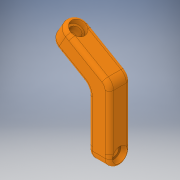
# Autodesk Inventor part: Link2
Saved by Autodesk Inventor 2019 (Build 230136000, 136)
## iProperties
Created: 2022-07-14
Part Number: Link2
Material: Generic
Document SubType Name: Modeling
Designer: zreik
Density: 1 g/cm^3
Appearance: Orange
d46: 10.000 mm
Author: zreik
Autodesk Inventor part; units mm, degrees
ref_plane "YZ Plane" through (0, 0, 0) normal (1, 0, 0) x (0, 1, 0)
ref_plane "XZ Plane" through (0, 0, 0) normal (0, 1, 0) x (-1, 0, 0)
ref_plane "XY Plane" through (0, 0, 0) normal (0, 0, 1) x (1, 0, 0)
sketch "Sketch1" plane through (0, 0, 0) normal (0, 0, 1) x (1, 0, 0)
  line L0 (44.0637, 0) -> (0, 0)
  line L1 (0, 0) -> (34.8308, 60.3287)
  line L2 (34.0637, 0) -> (34.0637, 22.1132)
  line L3 (31.5637, 26.4434) -> (19.3412, 33.5)
  line L4 (44.0637, 0) -> (44.0637, 27.8868)
  line L5 (41.5637, 32.2169) -> (24.3412, 42.1603)
  arc A0 (34.0637, 22.1132) -> (31.5637, 26.4434) centre (29.0637, 22.1132) ccw
  arc A1 (44.0637, 27.8868) -> (41.5637, 32.2169) centre (39.0637, 27.8868) ccw
  line L6 (24.3412, 42.1603) -> (19.3412, 33.5)
  line L7 (24.3412, 42.1603) -> (41.5637, 32.2169)
  line L8 (19.3412, 33.5) -> (31.5637, 26.4434)
  line L9 (34.0637, 0) -> (44.0637, 0)
  line L10 (44.0637, 0) -> (44.0637, 27.8868)
  line L11 (34.0637, 0) -> (44.0637, 0)
  line L12 (44.0637, 0) -> (44.0637, 27.8868)
  line L13 (41.5637, 32.2169) -> (24.3412, 42.1603)
  line L14 (24.3412, 42.1603) -> (19.3412, 33.5)
  line L15 (19.3412, 33.5) -> (31.5637, 26.4434)
  line L16 (34.0637, 22.1132) -> (34.0637, 0)
  point P0 (25, 43.3013)
  point P1 (34.0637, 25)
  dimension "d37" = 60
  dimension "d38" = 10
  dimension "d39" = 10
  dimension "d40" = 0
  dimension "d41" = 0
  dimension "d42" = 25
  dimension "d43" = 17
  dimension "d44" = 120
  dimension "d45" = 5
  constraints: 34 end point, 9 collinear, 6 point on line, 4 point on circle, 4 tangent, 2 centre point, 2 parallel, 1 coincident, 1 equal radius, 1 horizontal, 1 vertical
  measures "d37" angle of L1 L0
  measures "d38" distance between parallel lines of L3 L5
  measures "d39" distance between parallel lines of L4 L2
  measures "d40" distance from line of L1 L3.end
  measures "d41" distance from line of L1 L5.end
  measures "d42" distance of L2.start point (34.064, 25)
  measures "d43" distance of point (34.064, 25) L3.end
  measures "d44" angle of L2 L3
  measures "d45" radius of A0
extrude "Extrusion1" add sketch "Sketch1" along normal blind 10 contours L0 L2 A0 L3 L1 L5 A1 L4
ref_plane "Work Plane1" through (41.5637, 32.2169, 0) normal (0.5, 0.8660254, 0) x (-0.8660254, 0.5, 0)
sketch "Sketch2" plane through (41.5637, 32.2169, 0) normal (0.5, 0.8660254, 0) x (-0.8660254, 0.5, 0)
  circle A0 centre (19.8868, 5) radius 5
  line L0 (19.8868, 0) -> (19.8868, 10) projected
  line L1 (0, 10) -> (19.8868, 10) projected
  dimension "d5" = 10
  dimension "d47" = 0
  dimension "d48" = 5
  constraints: 1 centre point
  measures "d5" diameter of A0
  measures "d47" distance from line of L0 A0.centre
  measures "d48" distance from line of L1 A0.centre
extrude "Extrusion2" add sketch "Sketch2" against normal blind 10
ref_plane "Work Plane2" through (44.0637, 27.8868, 0) normal (1, 0, 0) x (0, 1, 0)
sketch "Sketch3" plane through (44.0637, 27.8868, 0) normal (1, 0, 0) x (0, 1, 0)
  circle A0 centre (-27.8868, 5) radius 5
  line L0 (43.3013, 10) -> (43.3013, 10) projected
  line L1 (-27.8868, 0) -> (-27.8868, 10) projected
  line L2 (-27.8868, 0) -> (0, 0) projected
  point P0 (5.6132, 10)
  dimension "d10" = 10
  dimension "d49" = 0
  dimension "d50" = 5
  constraints: 1 centre point, 1 horizontal alignment
  measures "d10" diameter of A0
  measures "d49" distance from line of L1 A0.centre
  measures "d50" distance from line of L2 A0.centre
extrude "Extrusion3" add sketch "Sketch3" against normal blind 10
sketch "Sketch4" plane through (36.5637, 23.5566, 0) normal (-0.5, -0.8660254, 0) x (0.8660254, -0.5, 0)
  circle A0 centre (-19.8868, 5) radius 2.5
  circle A1 centre (-19.8868, 5) radius 5 projected
  point P0 (-19.8868, 0)
  point P1 (-19.8868, 10)
  dimension "d15" = 5
  constraints: 1 centre point, 1 concentric
  measures "d15" diameter of A0
extrude "Extrusion4" cut sketch "Sketch4" along normal through all both and the other way through all contours A0
sketch "Sketch5" plane through (34.0637, 27.8868, 0) normal (-1, 0, 0) x (0, 0, 1)
  circle A0 centre (5, -27.8868) radius 2.5
  arc A1 (0, -27.8868) -> (10, -27.8868) centre (5, -27.8868) ccw projected
  dimension "d18" = 5
  constraints: 1 centre point, 1 concentric
  measures "d18" diameter of A0
extrude "Extrusion5" cut sketch "Sketch5" along normal through all both and the other way through all
sketch "Sketch6" plane through (41.5637, 32.2169, 0) normal (0.5, 0.8660254, 0) x (0.8660254, -0.5, 0)
  circle A0 centre (-19.8868, -5) radius 3.5
  circle A1 centre (-19.8868, -5) radius 2.5
  arc A2 (-19.8868, 0) -> (-19.8868, 0) centre (-19.8868, -5) ccw projected
  point P0 (0, -10)
  dimension "d21" = 5
  dimension "d22" = 7
  constraints: 2 centre point, 1 coincident, 2 other
  measures "d21" diameter of A1
  measures "d22" diameter of A0
extrude "Extrusion6" cut sketch "Sketch6" against normal blind 3 contours A0
sketch "Sketch7" plane through (36.5637, 23.5566, 0) normal (-0.5, -0.8660254, 0) x (0.8660254, -0.5, 0)
  circle A0 centre (-19.8868, 5) radius 3.5
  circle A1 centre (-19.8868, 5) radius 2.5
  arc A2 (-17.3868, 5) -> (-17.3868, 5) centre (-19.8868, 5) ccw projected
  point P0 (-19.8868, 0)
  dimension "d25" = 5
  dimension "d26" = 7
  constraints: 2 centre point, 1 coincident, 1 concentric
  measures "d25" diameter of A1
  measures "d26" diameter of A0
extrude "Extrusion7" cut sketch "Sketch7" along normal mid plane 6
sketch "Sketch8" plane through (34.0637, 27.8868, 0) normal (-1, 0, 0) x (0, 0, 1)
  circle A0 centre (5, -27.8868) radius 3.5
  circle A1 centre (5, -27.8868) radius 2.5
  arc A2 (7.5, -27.8868) -> (7.5, -27.8868) centre (5, -27.8868) ccw projected
  point P0 (0, -27.8868)
  dimension "d29" = 7
  dimension "d30" = 5
  constraints: 2 centre point, 1 coincident, 1 concentric
  measures "d29" diameter of A0
  measures "d30" diameter of A1
extrude "Extrusion8" cut sketch "Sketch8" along normal mid plane 6
sketch "Sketch9" plane through (44.0637, 27.8868, 0) normal (1, 0, 0) x (0, 0, -1)
  circle A0 centre (-5, -27.8868) radius 3.5
  circle A1 centre (-5, -27.8868) radius 2.5
  circle A2 centre (-5, -27.8868) radius 2.5 projected
  point P0 (0, -27.8868)
  dimension "d33" = 5
  dimension "d34" = 7
  constraints: 2 centre point, 1 coincident, 1 concentric
  measures "d33" diameter of A1
  measures "d34" diameter of A0
extrude "Extrusion9" cut sketch "Sketch9" against normal blind 3
fillet "Fillet1" radius 2 16 edges at (20.0111, 44.6603, 5) (32.9524, 37.1886, 0) (43.3938, 30.3868, 0) (44.0637, 13.9434, 0) (44.0637, -5, 5) (44.0637, 13.9434, 10) (43.3938, 30.3868, 10) (32.9524, 37.1886, 10) (33.3938, 24.6132, 10) (34.0637, 11.0566, 10) (34.0637, -5, 5) (34.0637, 11.0566, 0) (33.3938, 24.6132, 0) (25.4524, 29.9717, 0) (15.0111, 36, 5) (25.4524, 29.9717, 10)
equation "\"d38\" = d46"
equation "\"d39\" = d46"
equation "\"d3\" = width"
equation "\"d5\" = width"
equation "\"d48\" = 0.5 * width"
equation "\"d8\" = thickness"
equation "\"d10\" = width"
equation "\"d50\" = 0.5 * width"
equation "\"d13\" = thickness"
equation "\"thickness\" = thickness_1"
equation "\"width\" = width_1"
equation "\"d46\" = 10"
equation "\"thickness_1\" = 10"
equation "\"width_1\" = 10"
body "Solid1"
